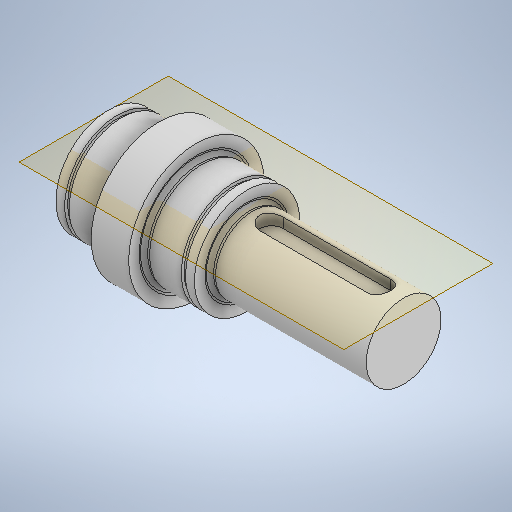
# Autodesk Inventor part: 1
Saved by Autodesk Inventor 2025.3 (Build 293356030, 356C)
## iProperties
Created: 2025-09-24
Part Number: 1
Material: Generisch
Document SubType Name: Modeling
Designer: tobia
Density: 1 g/cm^3
Appearance: Vorgabe
Author: tobia
Autodesk Inventor part; units mm, degrees
ref_plane "YZ Plane" through (0, 0, 0) normal (1, 0, 0) x (0, 1, 0)
ref_plane "XZ Plane" through (0, 0, 0) normal (0, 1, 0) x (-1, 0, 0)
sketch "Skizze8" plane through (0, 0, 0) normal (0, 0, 1) x (1, 0, 0)
  line L0 (0, 0) -> (0, 22.5)
  line L1 (0, 22.5) -> (21.65, 22.5)
  line L2 (21.65, 22.5) -> (21.65, 29)
  line L3 (21.65, 29) -> (37.65, 29)
  line L4 (37.65, 29) -> (37.65, 22.5)
  line L5 (37.65, 22.5) -> (59.3, 22.5)
  line L6 (59.3, 22.5) -> (59.3, 16)
  line L7 (59.3, 16) -> (126.3, 16)
  line L8 (126.3, 16) -> (126.3, 0)
  line L9 (126.3, 0) -> (0, 0)
  line L10 (-25.26, 0) -> (151.56, 0) projected
  constraints: 20 end point
revolve "Umdrehung7" add sketch "Skizze8" angle 360 about axis through (-10, 0, 0) along (1, 0, 0)
sketch "Skizze9" plane through (0, 0, 0) normal (0, 0, 1) x (1, 0, 0)
  line L0 (3.8, 21.25) -> (5.65, 21.25)
  line L1 (5.65, 21.25) -> (5.65, 22.5)
  line L2 (5.65, 22.5) -> (3.8, 22.5)
  line L3 (3.8, 22.5) -> (3.8, 21.25)
  line L4 (-25.26, 0) -> (151.56, 0) projected
  constraints: 8 end point, 2 parallel, 1 horizontal, 1 perpendicular
revolve "Umdrehung8" cut sketch "Skizze9" angle 360 about axis through (-10, 0, 0) along (1, 0, 0)
sketch "Skizze10" plane through (0, 0, 0) normal (0, 0, 1) x (1, 0, 0)
  line L0 (21.65, 24.5) -> (21.85, 23.7536)
  line L1 (20.2696, 22.2) -> (19.15, 22.5)
  line L2 (19.15, 22.5) -> (19.15, 24.5)
  line L3 (19.15, 24.5) -> (21.65, 24.5)
  arc A0 (20.2696, 22.2) -> (21.85, 23.7536) centre (20.7794, 23.262) ccw
  line L4 (-25.26, 0) -> (151.56, 0) projected
  constraints: 8 end point, 2 point on circle, 1 centre point
revolve "Umdrehung9" cut sketch "Skizze10" angle 360 about axis through (-10, 0, 0) along (1, 0, 0)
sketch "Skizze11" plane through (0, 0, 0) normal (0, 0, 1) x (1, 0, 0)
  line L0 (55.5, 21.25) -> (53.65, 21.25)
  line L1 (53.65, 21.25) -> (53.65, 22.5)
  line L2 (53.65, 22.5) -> (55.5, 22.5)
  line L3 (55.5, 22.5) -> (55.5, 21.25)
  line L4 (-25.26, 0) -> (151.56, 0) projected
  constraints: 8 end point, 2 parallel, 1 horizontal, 1 perpendicular
revolve "Umdrehung10" cut sketch "Skizze11" angle 360 about axis through (-10, 0, 0) along (1, 0, 0)
sketch "Skizze12" plane through (0, 0, 0) normal (0, 0, 1) x (1, 0, 0)
  line L0 (37.65, 24.5) -> (37.45, 23.7536)
  line L1 (39.0304, 22.2) -> (40.15, 22.5)
  line L2 (40.15, 22.5) -> (40.15, 24.5)
  line L3 (40.15, 24.5) -> (37.65, 24.5)
  arc A0 (37.45, 23.7536) -> (39.0304, 22.2) centre (38.5206, 23.262) ccw
  line L4 (-25.26, 0) -> (151.56, 0) projected
  constraints: 8 end point, 2 point on circle, 1 centre point
revolve "Umdrehung11" cut sketch "Skizze12" angle 360 about axis through (-10, 0, 0) along (1, 0, 0)
ref_plane "Arbeitsebene2" through (0, 0, 16) normal (0, 0, 1) x (1, 0, 0)
sketch "Skizze13" plane through (0, 0, 16) normal (0, 0, 1) x (1, 0, 0)
  line L0 (64.8, 0) -> (120.8, 0) construction
  line L1 (69.8, -5) -> (115.8, -5)
  line L2 (115.8, 5) -> (69.8, 5)
  arc A0 (69.8, 5) -> (69.8, -5) centre (69.8, 0) ccw
  arc A1 (115.8, -5) -> (115.8, 5) centre (115.8, 0) ccw
  point P0 (92.8, 0)
  constraints: 8 end point, 6 point on circle, 4 tangent, 2 centre point, 2 point on line, 1 midpoint, 1 parallel
extrude "Extrusion2" cut sketch "Skizze13" against normal blind 5
sketch "Skizze14" plane through (0, 0, 0) normal (0, 0, 1) x (1, 0, 0)
  line L0 (59.3, 18) -> (59.1, 17.2536)
  line L1 (60.6804, 15.7) -> (61.8, 16)
  line L2 (61.8, 16) -> (61.8, 18)
  line L3 (61.8, 18) -> (59.3, 18)
  arc A0 (59.1, 17.2536) -> (60.6804, 15.7) centre (60.1706, 16.762) ccw
  line L4 (-25.26, 0) -> (151.56, 0) projected
  constraints: 8 end point, 2 point on circle, 1 centre point
revolve "Umdrehung12" cut sketch "Skizze14" angle 360 about axis through (-10, 0, 0) along (1, 0, 0)
